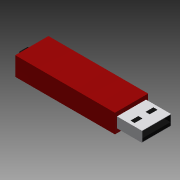
# Autodesk Inventor part: USB_Stick
Saved by Autodesk Inventor 2015 (Build 190159000, 159)
## iProperties
Created: 2013-02-21
Part Number: USB_Stick
Document SubType Name: Modeling
Density: 1 g/cm^3
Material: Generic
Appearance: Red
Autodesk Inventor part; units mm, degrees
ref_plane "YZ Plane" through (0, 0, 0) normal (1, 0, 0) x (0, 1, 0)
ref_plane "XZ Plane" through (0, 0, 0) normal (0, 1, 0) x (-1, 0, 0)
ref_plane "XY Plane" through (0, 0, 0) normal (0, 0, 1) x (1, 0, 0)
sketch "Sketch1" plane through (0, 0, 0) normal (0, 0, 1) x (1, 0, 0)
  line L0 (0, 6.3) -> (0, -6.3) projected
  line L1 (-33.6012, 0) -> (33.607, 0) projected
  line L2 (-24, 4.5) -> (24, 4.5)
  line L3 (24, 4.5) -> (24, -4.5)
  line L4 (24, -4.5) -> (-24, -4.5)
  line L5 (-24, -4.5) -> (-24, 4.5)
  dimension "d0" = 48
  dimension "d1" = 9
  constraints: 8 end point, 2 parallel, 1 horizontal, 1 perpendicular, 2 other
  measures "d0" distance of L2.start L2.end
  measures "d1" distance of L4.end L2.start
extrude "Legoblokje" add sketch "Sketch1" along normal mid plane 16
sketch "Sketch3" plane through (24, -4.5, 8) normal (1, 0, 0) x (0, 0, -1)
  line L0 (0, 9) -> (0, 0) projected
  line L1 (0, 0) -> (16, 0) projected
  line L2 (16, 0) -> (16, 9) projected
  line L3 (0, 9) -> (16, 9) projected
  line L4 (1, 7) -> (15, 7)
  line L5 (15, 7) -> (15, 2)
  line L6 (15, 2) -> (1, 2)
  line L7 (1, 2) -> (1, 7)
  point P0 (8, 4.5)
  dimension "d28" = 1
  dimension "d29" = 2
  dimension "d30" = 2
  dimension "d31" = 1
  dimension "d67" = 5
  constraints: 8 end point, 2 parallel, 1 horizontal, 1 perpendicular
  measures "d28" distance between parallel lines of L7 L0
  measures "d29" distance between parallel lines of L3 L4
  measures "d30" distance between parallel lines of L1 L6
  measures "d31" distance between parallel lines of L2 L5
  measures "d67" distance between parallel lines of L6 L4
extrude "USB" add sketch "Sketch3" along normal blind 12 contours L4 L5 L6 L7
sketch "Sketch4" plane through (36, -4.5, 8) normal (1, 0, 0) x (0, 0, -1)
  line L0 (15, 7) -> (15, 2) projected
  line L1 (1, 7) -> (15, 7) projected
  line L2 (1, 2) -> (1, 7) projected
  line L3 (15, 2) -> (1, 2) projected
  line L4 (1.2, 3.7) -> (14.8, 3.7)
  line L5 (14.8, 3.7) -> (14.8, 2.2)
  line L6 (14.8, 2.2) -> (1.2, 2.2)
  line L7 (1.2, 2.2) -> (1.2, 3.7)
  line L8 (1.2, 3.7) -> (14.8, 3.7)
  line L9 (14.8, 3.7) -> (14.8, 6.8)
  line L10 (14.8, 6.8) -> (1.2, 6.8)
  line L11 (1.2, 6.8) -> (1.2, 3.7)
  point P0 (8, 4.5)
  dimension "d34" = 0.2
  dimension "d35" = 0.2
  dimension "d36" = 0.2
  dimension "d37" = 1.5
  dimension "d38" = 0.2
  constraints: 16 end point, 4 parallel, 2 horizontal, 2 perpendicular
  measures "d34" distance between parallel lines of L2 L7
  measures "d35" distance between parallel lines of L3 L6
  measures "d36" distance between parallel lines of L0 L5
  measures "d37" distance between parallel lines of L6 L4
  measures "d38" distance between parallel lines of L1 L10
extrude "Afwerking USB" cut sketch "Sketch4" against normal blind 12 contours L11 L10 L9 L4
sketch "Sketch5" plane through (36, -4.5, 8) normal (1, 0, 0) x (0, 0, -1)
  line L0 (15, 2) -> (1, 2) projected
  line L1 (1.2, 3.7) -> (14.8, 3.7)
  line L2 (14.8, 3.7) -> (14.8, 2.2)
  line L3 (14.8, 2.2) -> (1.2, 2.2)
  line L4 (1.2, 2.2) -> (1.2, 3.7)
  point P0 (8, 4.5)
  dimension "d41" = 0.2
  constraints: 8 end point, 2 parallel, 1 horizontal, 1 perpendicular
  measures "d41" distance between parallel lines of L0 L3
extrude "Afwerking" cut sketch "Sketch5" against normal blind 0.01
sketch "Sketch6" plane through (24, 2.5, 7) normal (0, 1, 0) x (1, 0, 0)
  line L0 (0, 14) -> (12, 14) projected
  line L1 (0, 0) -> (0, 14) projected
  line L2 (0, 0) -> (12, 0) projected
  line L3 (5, 12.5) -> (7, 12.5)
  line L4 (7, 12.5) -> (7, 8.75)
  line L5 (7, 8.75) -> (5, 8.75)
  line L6 (5, 8.75) -> (5, 12.5)
  line L7 (5, 5.25) -> (7, 5.25)
  line L8 (7, 5.25) -> (7, 1.5)
  line L9 (7, 1.5) -> (5, 1.5)
  line L10 (5, 1.5) -> (5, 5.25)
  point P0 (-24, 7)
  dimension "d44" = 5
  dimension "d45" = 5
  dimension "d46" = 1.5
  dimension "d47" = 1.5
  dimension "d48" = 3.5
  dimension "d49" = 2
  dimension "d50" = 2
  dimension "d51" = 3.75
  dimension "d52" = 3.75
  constraints: 16 end point, 4 parallel, 2 horizontal, 2 perpendicular
  measures "d44" distance between parallel lines of L1 L6
  measures "d45" distance between parallel lines of L1 L10
  measures "d46" distance between parallel lines of L0 L3
  measures "d47" distance between parallel lines of L2 L9
  measures "d48" distance between parallel lines of L7 L5
  measures "d49" distance between parallel lines of L10 L8
  measures "d50" distance between parallel lines of L6 L4
  measures "d51" distance between parallel lines of L3 L5
  measures "d52" distance between parallel lines of L9 L7
extrude "Afwerking bovenkant" cut sketch "Sketch6" against normal blind 0.1
sketch "Sketch7" plane through (-24, -4.5, 8) normal (-1, 0, 0) x (0, 0, 1)
  line L0 (-10, 5.5) -> (-6, 5.5)
  line L1 (-6, 5.5) -> (-6, 3.5)
  line L2 (-6, 3.5) -> (-10, 3.5)
  line L3 (-10, 3.5) -> (-10, 5.5)
  point P0 (-8, 4.5)
  dimension "d55" = 1
  dimension "d56" = 1
  dimension "d57" = 2
  dimension "d58" = 2
  constraints: 8 end point, 2 parallel, 1 horizontal, 1 perpendicular
  measures "d55" distance from line of L0 point (-8, 4.5)
  measures "d56" distance from line of point (-8, 4.5) L2
  measures "d57" distance from line of point (-8, 4.5) L3
  measures "d58" distance from line of L1 point (-8, 4.5)
extrude "Achterkant afwerking" add sketch "Sketch7" along normal blind 4
sketch "Sketch8" plane through (-24, 1, 2) normal (0, 1, 0) x (1, 0, 0)
  circle A0 centre (-2, 2) radius 1.5
  point P0 (24, 2)
  dimension "d61" = 3
  constraints: 1 centre point
  measures "d61" diameter of A0
extrude "afwerking gat" cut sketch "Sketch8" against normal through all
body "Solid1"
